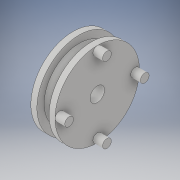
# Autodesk Inventor part: SpoolWindDriver
Saved by Autodesk Inventor 2019 (Build 230136000, 136)
## iProperties
Created: 2019-01-14
Part Number: SpoolWindDriver
Material: Generic
Document SubType Name: Modeling
Designer: Kepler
Density: 1 g/cm^3
Appearance: Default
Author: Kepler
Autodesk Inventor part; units mm, degrees
ref_plane "YZ Plane" through (0, 0, 0) normal (1, 0, 0) x (0, 1, 0)
ref_plane "XZ Plane" through (0, 0, 0) normal (0, 1, 0) x (-1, 0, 0)
ref_plane "XY Plane" through (0, 0, 0) normal (0, 0, 1) x (1, 0, 0)
sketch "Sketch3" plane through (0, 0, 0) normal (0, 0, 1) x (1, 0, 0)
  line L0 (0, 0) -> (0, 14.4)
  line L1 (0, 17.4) -> (10, 17.4)
  line L2 (10, 14.4) -> (10, 0)
  line L3 (10, 0) -> (7.5, 0)
  line L4 (7.5, 0) -> (7.5, 3)
  line L5 (7.5, 3) -> (2.5, 3)
  line L6 (2.5, 3) -> (2.5, 0)
  line L7 (2.5, 0) -> (0, 0)
  line L8 (0, 14.4) -> (10, 14.4)
  dimension "d18" = 3.6
  dimension "d10" = 17.4
  dimension "d11" = 10
  dimension "d12" = 2.5
  dimension "d13" = 3
  dimension "d14" = 5
  dimension "d24" = 6
  dimension "d25" = 14.4
  constraints: 18 end point, 6 perpendicular, 1 horizontal, 1 parallel, 1 point on line, 1 vertical
  measures "d10" distance of L0.start L1.start
  measures "d11" distance of L1.start L1.end
  measures "d12" distance of L2.end L3.end
  measures "d13" distance of L3.end L4.end
  measures "d14" distance of L4.end L5.end
  measures "d24" diameter of L8 L1
  measures "d25" distance between parallel lines of L3 L8
sketch "Sketch4" plane through (0, 0, 0) normal (0, 0, 1) x (1, 0, 0)
  point P0 (0, 0)
revolve "Revolution1" add sketch "Sketch3" angle 360 about axis through (0, 17.4, 0) along (1, 0, 0)
sketch "Sketch5" plane through (10, 17.4, 0) normal (1, 0, 0) x (0, 0, -1)
  circle A0 centre (15.6, 0) radius 1.8
  circle A1 centre (0, 15.6) radius 1.8
  circle A2 centre (-15.6, 0) radius 1.8
  circle A3 centre (0, -15.6) radius 1.8
  circle A4 centre (0, 0) radius 17.4 projected
  point P0 (0, -17.4)
  dimension "d16" = 3.6
  dimension "d17" = 3.6
  dimension "d18" = 3.6
  dimension "d19" = 3.6
  constraints: 4 centre point, 1 vertical alignment, 5 other
  measures "d16" diameter of A0
  measures "d17" diameter of A1
  measures "d18" diameter of A2
  measures "d19" diameter of A3
extrude "Extrusion3" add sketch "Sketch5" along normal blind 4 contours A0 | A1 | A2 | A3
body "Solid2"
